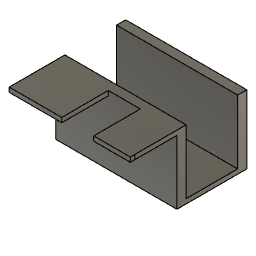
soporteInfraRed (Autodesk Fusion 360 design; units mm, degrees)
Autodesk Fusion 360 part; units mm, degrees
sketch "Boceto1" plane through (0, 0, 0) normal (0, 0, 1) x (1, 0, 0)
  line L0 (0.2278, 20.1586) -> (40.2278, 20.1586)
  line L1 (40.2278, 20.1586) -> (40.2278, 8.8586)
  line L2 (40.2278, 8.8586) -> (0.2278, 8.8586)
  line L3 (0.2278, 8.8586) -> (0.2278, 20.1586)
  line L4 (0.2278, 20.1586) -> (40.2278, 20.1586)
  line L5 (40.2278, 20.1586) -> (40.2278, 24.1586)
  line L6 (40.2278, 24.1586) -> (0.2278, 24.1586)
  line L7 (0.2278, 24.1586) -> (0.2278, 20.1586)
  line L8 (0.2278, 8.8586) -> (40.2278, 8.8586)
  line L9 (40.2278, 8.8586) -> (40.2278, 4.8586)
  line L10 (40.2278, 4.8586) -> (0.2278, 4.8586)
  line L11 (0.2278, 4.8586) -> (0.2278, 8.8586)
  dimension "d1" = 40
  dimension "d2" = 11.3
  dimension "d3" = 4
  dimension "d4" = 40
  dimension "d5" = 4
  constraint horizontal L0
  constraint vertical L1
  constraint horizontal L2
  constraint vertical L3
  constraint horizontal L4
  constraint vertical L5
  constraint horizontal L6
  constraint vertical L7
  constraint horizontal L8
  constraint vertical L9
  constraint horizontal L10
  constraint vertical L11
  measures "d1" distance of L0.start L0.end
  measures "d2" distance of L0.start L2.end
  measures "d3" distance of L0.start L6.end
  measures "d4" distance of L2.end L1.end
  measures "d5" distance of L2.end L10.end
extrude "Extruir1" add sketch "Boceto1" along normal blind 15
extrude "Extruir2" cut sketch "Boceto1" along normal blind 14 contours L0 L1 L2 L3 L4 L8
sketch "Boceto2" plane through (0, 24.1586, 0) normal (0, 1, 0) x (-1, 0, 0)
  line L0 (-40.2278, 0) -> (-0.2278, 0)
  line L1 (-0.2278, 0) -> (-0.2278, 15)
  line L2 (-0.2278, 15) -> (-40.2278, 15)
  line L3 (-40.2278, 15) -> (-40.2278, 0)
  line L4 (-40.2278, 0) -> (-0.2278, 0)
  line L5 (-0.2278, 0) -> (-0.2278, 1)
  line L6 (-0.2278, 1) -> (-40.2278, 1)
  line L7 (-40.2278, 1) -> (-40.2278, 0)
  dimension "d10" = 40
  dimension "d11" = 1
  constraint horizontal L4
  constraint vertical L5
  constraint horizontal L6
  constraint vertical L7
  constraint coincident L0.start L3.end
  measures "d10" distance of L0.start L0.end
  measures "d11" distance of L0.start L6.end
extrude "Extruir3" add sketch "Boceto2" along normal blind 10.2 contours L0 L1 L3 L4 L5 L6 L7
sketch "Boceto3" plane through (0, 0, 1) normal (0, 0, 1) x (-1, 0, 0)
  line L0 (-0.2278, -24.1586) -> (-40.2278, -24.1586)
  line L1 (-40.2278, -24.1586) -> (-40.2278, -34.3586)
  line L2 (-40.2278, -34.3586) -> (-0.2278, -34.3586)
  line L3 (-0.2278, -34.3586) -> (-0.2278, -24.1586)
  line L4 (-0.2278, -24.1586) -> (-11.7278, -24.1586)
  line L5 (-11.7278, -24.1586) -> (-11.7278, -34.3586)
  line L6 (-11.7278, -34.3586) -> (-0.2278, -34.3586)
  line L7 (-0.2278, -34.3586) -> (-0.2278, -24.1586)
  line L8 (-11.7278, -24.1586) -> (-18.7278, -24.1586)
  line L9 (-18.7278, -24.1586) -> (-18.7278, -34.3586)
  line L10 (-18.7278, -34.3586) -> (-11.7278, -34.3586)
  line L11 (-11.7278, -34.3586) -> (-11.7278, -24.1586)
  line L12 (-18.7278, -24.1586) -> (-26.7278, -24.1586)
  line L13 (-26.7278, -24.1586) -> (-26.7278, -34.3586)
  line L14 (-26.7278, -34.3586) -> (-18.7278, -34.3586)
  line L15 (-18.7278, -34.3586) -> (-18.7278, -24.1586)
  dimension "d14" = 11.5
  dimension "d15" = 10.2
  dimension "d16" = 7
  dimension "d17" = 10.2
  dimension "d18" = 8
  dimension "d19" = 10.2
  constraint horizontal L4
  constraint vertical L5
  constraint horizontal L6
  constraint vertical L7
  constraint coincident L0.start L3.end
  constraint horizontal L8
  constraint vertical L9
  constraint horizontal L10
  constraint vertical L11
  constraint horizontal L12
  constraint vertical L13
  constraint horizontal L14
  constraint vertical L15
  measures "d14" distance of L0.start L4.end
  measures "d15" distance of L0.start L2.end
  measures "d16" distance of L4.end L8.end
  measures "d17" distance of L4.end L5.end
  measures "d18" distance of L8.end L12.end
  measures "d19" distance of L8.end L9.end
extrude "Extruir4" cut sketch "Boceto3" against normal blind 20 contours L0 L2 L5 L8 L9 L10 L11 L15
sketch "Boceto4" plane through (0, 0, 1) normal (0, 0, 1) x (-1, 0, 0)
  line L0 (-26.7493, -34.2964) -> (-43.5631, -34.2964)
  line L1 (-43.5631, -34.2964) -> (-43.5631, -0.0955)
  line L2 (-43.5631, -0.0955) -> (-26.7493, -0.0955)
  line L3 (-26.7493, -0.0955) -> (-26.7493, -34.2964)
  constraint horizontal L0
  constraint vertical L1
  constraint horizontal L2
  constraint vertical L3
extrude "Extruir5" cut sketch "Boceto4" along normal blind 40 and the other way blind 40
sketch "Boceto5" plane through (0, 34.3586, 0) normal (0, 1, 0) x (-1, 0, 0)
  line L0 (-18.7278, 0) -> (-18.7278, 1)
  line L1 (-18.7278, 1) -> (-40.2278, 1)
  line L2 (-40.2278, 1) -> (-40.2278, 0)
  line L3 (-40.2278, 0) -> (-18.7278, 0)
  line L4 (-40.2278, 1) -> (-26.6927, 1)
  line L5 (-26.6927, 1) -> (-26.6927, 0)
  line L6 (-26.6927, 0) -> (-40.2278, 0)
  line L7 (-40.2278, 0) -> (-40.2278, 1)
  constraint horizontal L4
  constraint vertical L5
  constraint horizontal L6
  constraint vertical L7
  constraint coincident L3 L5.end
  constraint coincident L1.end L2.start
extrude "Extruir6" cut sketch "Boceto5" against normal blind 3 contours L1 L2 L3 L4 L5 L6 L7
extrude "Extruir7" add 1 faces at (26.6927, 33.3586, 0.6667) along direction (1, 0, 0) blind 0.057
extrude "Extruir8" cut 1 faces at (17.9088, 4.8586, 5) along direction (0, 1, 0) blind 2
extrude "Extruir9" cut 1 faces at (12.9016, 24.1586, 10.3333) along direction (0, -1, 0) blind 2
extrude "Extruir10" cut 2 faces at (21.4018, 34.3586, 0.6667) (7.8944, 34.3586, 0.6667) along direction (0, -1, 0) blind 2
move_body "Desplazar1" bodies 1 to x (1, 0, 0) y (0, -1, 0) z (0, 0, -1) at (0, 13.7172, 0)
